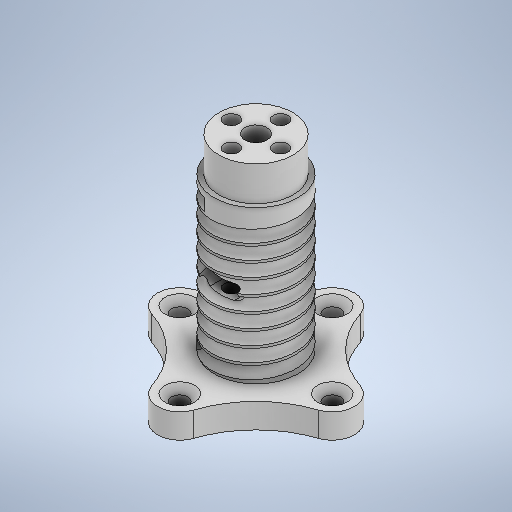
# Autodesk Inventor part: Small_drum
Saved by Autodesk Inventor 2025.2 (Build 292293000, 293)
## iProperties
Created: 2025-04-05
Part Number: Small_drum
Material: Generic
Document SubType Name: Modeling
Designer: Bruno
Density: 1 g/cm^3
Appearance: Default
Mass: 8.9379 g
Surface Area: 66.8314 cm^2
Volume: 8.9379 cm^3
Author: Bruno
## iProperties of the stored document Small_drum_3DPrint.ipt
Created: 2025-04-25
Part Number: Small_drum_3DPrint
Material: Generic
Document SubType Name: Modeling
Designer: Bruno
Density: 1 g/cm^3
Appearance: Default
Author: Bruno
Autodesk Inventor part; units mm, degrees
ref_plane "YZ Plane" through (0, 0, 0) normal (1, 0, 0) x (0, 1, 0)
ref_plane "XZ Plane" through (0, 0, 0) normal (0, 1, 0) x (-1, 0, 0)
sketch "Sketch1" plane through (0, 0, 0) normal (0, 1, 0) x (-1, 0, 0)
  arc A0 (16.9224, -4.2693) -> (16.9224, 4.2693) centre (15.5, 0) ccw
  arc A1 (4.2693, 16.9224) -> (-4.2693, 16.9224) centre (0, 15.5) ccw
  arc A2 (-4.2693, -16.9224) -> (4.2693, -16.9224) centre (0, -15.5) ccw
  arc A3 (-16.9224, 4.2693) -> (-16.9224, -4.2693) centre (-15.5, 0) ccw
  arc A4 (4.2693, 16.9224) -> (16.9224, 4.2693) centre (23.244, 23.244) ccw
  line L0 (0, -32.5415) -> (0, 32.5415) projected
  line L1 (32.5415, 0) -> (-32.5415, 0) projected
  arc A5 (16.9224, -4.2693) -> (4.2693, -16.9224) centre (23.244, -23.244) ccw
  arc A6 (-16.9224, 4.2693) -> (-4.2693, 16.9224) centre (-23.244, 23.244) ccw
  arc A7 (-4.2693, -16.9224) -> (-16.9224, -4.2693) centre (-23.244, -23.244) ccw
  line L2 (0, 15.5) -> (0, -15.5)
  point P0 (0, 0)
  dimension "d0" = 9
  dimension "d1" = 9
  dimension "d2" = 9
  dimension "d3" = 9
  dimension "d5" = 31
  dimension "d6" = 31
  dimension "d10" = 15.5
  dimension "d11" = 15.5
  dimension "d12" = 20
  dimension "d13" = 20
  dimension "d14" = 20
  dimension "d15" = 20
  constraints: 16 point on circle, 8 centre point, 8 tangent, 4 point on line, 2 end point, 1 vertical
  measures "d0" diameter of A1
  measures "d1" diameter of A0
  measures "d2" diameter of A2
  measures "d3" diameter of A3
  measures "d5" distance of L2.end L2.start
  measures "d6" distance of A3.centre A0.centre
  measures "d10" distance from line of L2.end L1
  measures "d11" distance from line of L2 A0.centre
  measures "d12" radius of A6
  measures "d13" radius of A7
  measures "d14" radius of A5
  measures "d15" radius of A4
extrude "Extrusion1" add sketch "Sketch1" along normal blind 5
sketch "Sketch2" plane through (0, 5, 0) normal (0, 1, 0) x (1, 0, 0)
  circle A0 centre (0, 0) radius 8.5
  dimension "d18" = 17
  constraints: 1 centre point, 1 coincident
  measures "d18" diameter of A0
extrude "Extrusion2" add sketch "Sketch2" along normal blind 38
sketch "Sketch3" plane through (0, 43, 0) normal (0, 1, 0) x (1, 0, 0)
  circle A0 centre (0, 0) radius 7.5
  circle A1 centre (0, 0) radius 8.5 projected
  dimension "d21" = 15
  constraints: 1 centre point, 1 coincident
  measures "d21" diameter of A0
extrude "Extrusion3" cut sketch "Sketch3" against normal blind 7
ref_plane "Work Plane1" through (0, 5, 0) normal (-0.7071068, 0, -0.7071068) x (0, -1, 0)
sketch "Sketch6" plane through (0, 5, 0) normal (-0.7071068, 0, -0.7071068) x (0, -1, 0)
  circle A0 centre (-1.25, 8.5) radius 1.25
  line L0 (0, 15.4602) -> (0, 8.9471) projected
  line L1 (0, 8.5) -> (-31, 8.5) projected
  point P0 (5, 0)
  point P1 (0, 14.9848)
  dimension "d34" = 2.5
  constraints: 1 centre point, 1 point on line, 1 tangent
  measures "d34" diameter of A0
coil "Coil2" sketch "Sketch6" operation cut axis through (0, 5, 0) along (0, 1, 0) pitch 3 turns 9.083333 hand right
sketch "Sketch7" plane through (0, 0, 0) normal (0, 0, 1) x (1, 0, 0)
  arc A0 (-2.5, 21.375) -> (-2.5, 18.375) centre (-2.5, 19.875) ccw
  arc A1 (2.5, 18.375) -> (2.5, 21.375) centre (2.5, 19.875) ccw
  line L0 (-2.5, 21.375) -> (2.5, 21.375)
  line L1 (-2.5, 18.375) -> (2.5, 18.375)
  line L2 (-8.5, 36) -> (8.5, 36) projected
  line L3 (4.2693, 5) -> (-4.2693, 5) projected
  line L4 (1.0707, 19.875) -> (16.4612, 19.875)
  line L5 (0, 36) -> (0, 5)
  point P0 (0, 0)
  point P1 (-2.2, 34.75)
  dimension "d45" = 5
  dimension "d46" = 1.5
  dimension "d47" = 1.5
  dimension "d49" = 14.875
  dimension "d50" = 3
  dimension "d51" = 5
  constraints: 8 end point, 4 point on circle, 3 horizontal, 2 centre point, 2 midpoint, 2 tangent, 1 horizontal alignment
  measures "d45" distance of L0.start L0.end
  measures "d46" radius of A0
  measures "d47" radius of A1
  measures "d49" distance from line of L4 point (-2.2, 34.75)
  measures "d50" diameter of L0 L4
  measures "d51" diameter of A0.centre L5
extrude "Extrusion4" cut sketch "Sketch7" along normal through all both and the other way through all
sketch "Sketch8" plane through (0, 0, 0) normal (0, -1, 0) x (1, 0, 0)
  circle A0 centre (0, 0) radius 2.25
  circle A1 centre (-5, 0) radius 2.75
  circle A2 centre (0, -5) radius 2.75
  circle A3 centre (5, 0) radius 2.75
  circle A4 centre (0, 5) radius 2.75
  arc A5 (-5.6379, 2.675) -> (-2.675, 5.6379) centre (-6.5659, 6.5659) ccw
  arc A6 (2.675, 5.6379) -> (5.6379, 2.675) centre (6.5659, 6.5659) ccw
  arc A7 (5.6379, -2.675) -> (2.675, -5.6379) centre (6.5659, -6.5659) ccw
  arc A8 (-2.675, -5.6379) -> (-5.6379, -2.675) centre (-6.5659, -6.5659) ccw
  dimension "d54" = 4.5
  dimension "d55" = 5.5
  dimension "d58" = 360
  dimension "d60" = 4
  dimension "d61" = 4
  dimension "d62" = 4
  dimension "d63" = 4
  constraints: 16 point on circle, 9 centre point, 9 tangent, 1 coincident, 1 horizontal alignment, 9 other
  measures "d54" diameter of A0
  measures "d55" diameter of A1
  measures "d60" radius of A5
  measures "d61" radius of A6
  measures "d62" radius of A7
  measures "d63" radius of A8
extrude "Extrusion5" cut sketch "Sketch8" against normal blind 3.5
sketch "Sketch9" plane through (0, 3.5, 0) normal (0, -1, 0) x (1, 0, 0)
  circle A0 centre (0, 5) radius 1.5
  arc A1 (2.675, 5.6379) -> (-2.675, 5.6379) centre (0, 5) ccw projected
  circle A2 centre (-5, 0) radius 1.5
  circle A3 centre (0, -5) radius 1.5
  circle A4 centre (5, 0) radius 1.5
  point P0 (0, 0)
  dimension "d66" = 3
  dimension "d69" = 360
  constraints: 4 centre point, 1 concentric, 9 other
  measures "d66" diameter of A0
extrude "Extrusion6" cut sketch "Sketch9" against normal through all
sketch "Sketch10" plane through (0, 3.5, 0) normal (0, -1, 0) x (1, 0, 0)
  circle A0 centre (0, 0) radius 2.25
  dimension "d73" = 4.5
  constraints: 1 centre point, 1 coincident
  measures "d73" diameter of A0
extrude "Extrusion7" cut sketch "Sketch10" against normal blind 4
sketch "Sketch11" plane through (0, 5, 0) normal (0, 1, 0) x (1, 0, 0)
  arc A0 (16.9224, -4.2693) -> (16.9224, 4.2693) centre (15.5, 0) ccw projected
  circle A1 centre (15.5, 0) radius 1.65
  circle A2 centre (0, 15.5) radius 1.65
  circle A3 centre (-15.5, 0) radius 1.65
  circle A4 centre (0, -15.5) radius 1.65
  point P0 (0, 0)
  dimension "d76" = 3.3
  dimension "d79" = 360
  constraints: 4 centre point, 1 coincident, 9 other
  measures "d76" diameter of A1
extrude "Extrusion8" cut sketch "Sketch11" against normal through all
chamfer "Chamfer1" distance 1.35 angle 45 4 edges at (-1.65, 5, 15.5) (-17.15, 5, 0) (13.85, 5, 0) (-1.65, 5, -15.5)
sketch "Sketch12" plane through (0, 43, 0) normal (0, 1, 0) x (1, 0, 0)
  circle A0 centre (0, 0) radius 2.225
  dimension "d86" = 4.45
  constraints: 1 centre point, 1 coincident
  measures "d86" diameter of A0
extrude "Extrusion9" cut sketch "Sketch12" against normal blind 7.5
sketch "Sketch15" plane through (0, 3.5, 0) normal (0, -1, 0) x (1, 0, 0)
  circle A0 centre (0, 0) radius 2.25 projected
  circle A1 centre (5, 0) radius 1.5 projected
  circle A2 centre (-5, 0) radius 1.5 projected
  circle A3 centre (0, -5) radius 1.5 projected
  circle A4 centre (0, 5) radius 1.5 projected
  arc A5 (-2.675, -5.6379) -> (-5.6379, -2.675) centre (-6.5659, -6.5659) ccw projected
  arc A6 (-2.675, -5.6379) -> (2.675, -5.6379) centre (0, -5) ccw projected
  arc A7 (5.6379, -2.675) -> (2.675, -5.6379) centre (6.5659, -6.5659) ccw projected
  arc A8 (5.6379, -2.675) -> (5.6379, 2.675) centre (5, 0) ccw projected
  arc A9 (2.675, 5.6379) -> (5.6379, 2.675) centre (6.5659, 6.5659) ccw projected
  arc A10 (2.675, 5.6379) -> (-2.675, 5.6379) centre (0, 5) ccw projected
  arc A11 (-5.6379, 2.675) -> (-2.675, 5.6379) centre (-6.5659, 6.5659) ccw projected
  arc A12 (-5.6379, 2.675) -> (-5.6379, -2.675) centre (-5, 0) ccw projected
  line L0 (-7.6905, -0.5691) -> (0.5691, 7.6905)
  circle A13 centre (0, 5) radius 1.5 projected
  circle A14 centre (-5, 0) radius 1.5 projected
  line L1 (-5.5704, -2.6917) -> (2.6917, 5.5704)
  line L2 (0, 0) -> (1.0668, 1.0668) construction
  line L3 (-0.5691, -7.6905) -> (7.6905, 0.5691)
  line L4 (-2.6917, -5.5704) -> (5.5704, 2.6917)
  point P0 (7.6905, 0.5691)
  point P1 (5.5704, 2.6917)
  constraints: 10 end point, 4 point on circle, 4 symmetric about line, 4 tangent, 1 parallel
extrude "Extrusion10" add sketch "Sketch15" along normal blind 0.2 contours A0 L4 L1 | A0 L1 A9 L4 | A0 L4 A5 L1 | L0 A12 A11 A10 | L3 A8 A7 A6
sketch "Sketch16" plane through (2.5, 21.375, -8.124) normal (0, -1, 0) x (1, 0, 0)
  line L0 (-5, 0.6307) -> (-5, 14.9322) projected
  line L1 (0, 15.0054) -> (0, 0) projected
  line L2 (-5, 14.624) -> (0, 14.624)
  circle A0 centre (-2.5, 13.124) radius 1.5 projected
  line L3 (-5, 11.624) -> (0, 11.624)
  line L4 (-5, 4.624) -> (0, 4.624)
  line L5 (0, 1.624) -> (-5, 1.624)
  circle A1 centre (-2.5, 3.124) radius 1.5 projected
  circle A2 centre (-2.5, 3.124) radius 1.5 projected
  circle A3 centre (-2.5, 13.124) radius 1.5 projected
  line L6 (-5, 0.6307) -> (-5, 14.9322) projected
  arc A4 (-2.5, -0.376) -> (0, 0) centre (-2.5, 8.124) ccw projected
  line L7 (0, 15.0054) -> (0, 0) projected
  point P0 (-2.5, 11.624)
  point P1 (-2.5, 14.624)
  point P2 (-2.5, 1.624)
  point P3 (-2.5, 4.624)
  constraints: 8 end point, 8 point on line, 4 horizontal, 4 tangent, 2 other
extrude "Extrusion11" cut sketch "Sketch16" against normal blind 0.2 contours L0 L4 A1 L5 | A1 L4 L1 L5 | L0 L2 A0 L3 | A0 L2 L1 L3
body "Solid1"
